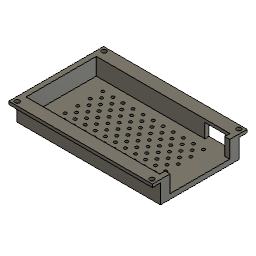
Portable+Battery+Case (Autodesk Fusion 360 design; units mm, degrees)
Autodesk Fusion 360 part; units mm, degrees
note: some values were not read from the file. Set by a fixed rule: which sketch regions a step uses.
sketch "Sketch1" plane through (0, 0, 0) normal (0, 1, 0) x (1, 0, 0)
  line L0 (-66.4, 34.9) -> (66.4, 34.9)
  line L1 (66.4, 34.9) -> (66.4, -34.9)
  line L2 (66.4, -34.9) -> (-66.4, -34.9)
  line L3 (-66.4, -34.9) -> (-66.4, 34.9)
  line L4 (-71.4, -39.15) -> (71.4, -39.15)
  line L5 (71.4, 39.15) -> (71.4, -39.15)
  line L6 (0, 0) -> (-71.6, 0) construction
  line L7 (-71.4, 39.15) -> (71.4, 39.15)
  line L8 (-71.4, 39.15) -> (-71.4, -39.15)
  dimension "d1" = 69.8
  dimension "d2" = 132.8
  dimension "d3" = 66.4
  dimension "d4" = 34.9
  dimension "d40" = 4.25
  dimension "d46" = 4.25
  dimension "d47" = 5
  dimension "d63" = 5
  constraint horizontal L0
  constraint vertical L1
  constraint horizontal L2
  constraint vertical L3
  constraint coincident L6.start origin
  constraint horizontal L6
  constraint perpendicular L5 L7
  constraint perpendicular L4 L5
  constraint perpendicular L7 L8
  measures "d1" distance of L0.start L2.end
  measures "d2" distance of L0.start L0.end
  measures "d3" distance of L6.start L3
  measures "d4" distance of L6.start L0
  measures "d40" distance of L2 L4
  measures "d46" distance of L0 L7
  measures "d47" distance of L1 L5
  measures "d63" distance of L3 L8
extrude "Extrude1" add sketch "Sketch1" along normal blind 5 contours L0 L1 L2 L3
extrude "Extrude2" add sketch "Sketch1" along normal blind 22.018
sketch "Sketch3" plane through (0, 22.018, 0) normal (0, 1, 0) x (-1, 0, 0)
  line L0 (-66.4, 34.9) -> (66.4, 34.9)
  line L1 (66.4, 34.9) -> (66.4, -34.9)
  line L2 (66.4, -34.9) -> (-66.4, -34.9)
  line L3 (-66.4, -34.9) -> (-66.4, 34.9)
  line L4 (62.4, -47.15) -> (-71.4, -47.15)
  line L5 (-71.4, -47.15) -> (-71.4, 47.15)
  line L6 (-71.4, 47.15) -> (71.4, 47.15)
  circle A0 centre (66.9, -43.15) radius 2.25
  circle A1 centre (-66.9, -43.15) radius 2.25
  circle A2 centre (-66.9, 43.15) radius 2.25
  circle A3 centre (66.9, 43.15) radius 2.25
  line L7 (71.4, 39.15) -> (-71.4, 39.15)
  line L8 (-71.4, 39.15) -> (-71.4, -39.15)
  line L9 (-71.4, -39.15) -> (71.4, -39.15)
  line L10 (62.4, -47.15) -> (71.4, -47.15)
  line L11 (71.4, 39.15) -> (71.4, 47.15)
  line L12 (71.4, -39.15) -> (71.4, 39.15)
  line L13 (71.4, -47.15) -> (71.4, -39.15)
  point P0 (-71.4, 0)
  point P1 (71.4, 39.15)
  dimension "d23" = 4.5
  dimension "d24" = 4
  dimension "d25" = 4.5
  dimension "d26" = 4.5
  dimension "d27" = 4
  dimension "d29" = 4.5
  dimension "d30" = 4.5
  dimension "d31" = 4
  dimension "d32" = 4.5
  dimension "d50" = 9
  dimension "d51" = 4.5
  dimension "d52" = 4
  dimension "d64" = 8
  dimension "d65" = 8
  dimension "d66" = 4.5
  constraint horizontal L4
  constraint vertical L5
  constraint horizontal L6
  constraint midpoint L5 P0
  constraint coincident L8.end L5
  constraint coincident P1 L7.start
  constraint perpendicular L6 L11
  constraint perpendicular L9 L13
  constraint coincident L9.end L12.start
  constraint perpendicular L10 L13
  measures "d23" diameter of A0
  measures "d24" distance of L4 A1.centre
  measures "d25" distance of L5 A1.centre
  measures "d26" diameter of A1
  measures "d27" distance of L6 A3.centre
  measures "d29" diameter of A3
  measures "d30" distance of L5 A2.centre
  measures "d31" distance of L6 A2.centre
  measures "d32" diameter of A2
  measures "d50" distance of L4.start L10.end
  measures "d51" distance of A3.centre L11
  measures "d52" distance of A0.centre L10
  measures "d64" distance of L6 L7
  measures "d65" distance of L10.end L9.end
  measures "d66" distance of A0.centre L13
extrude "Extrude4" add sketch "Sketch3" against normal blind 3 contours L4 L5 L9 L10 L13 | L5 L6 L7 L11
sketch "Sketch2" plane through (71.4, 0, 0) normal (1, 0, 0) x (0, 0, -1)
  line L0 (39.65, 0) -> (39.65, 18.75)
  line L1 (-34.65, 5) -> (34.65, 5)
  line L2 (34.65, 5) -> (-34.65, 5)
  line L3 (-29.65, 22.018) -> (29.65, 22.018)
  line L4 (29.65, 22.018) -> (29.65, 5)
  line L5 (29.65, 5) -> (-29.65, 5)
  line L6 (-29.65, 5) -> (-29.65, 22.018)
  line L7 (-39.15, 0) -> (39.15, 0)
  line L8 (39.15, 19.018) -> (47.15, 19.018)
  line L9 (47.15, 19.018) -> (47.15, 22.018)
  line L10 (47.15, 22.018) -> (-47.15, 22.018)
  line L11 (-47.15, 22.018) -> (-47.15, 19.018)
  line L12 (-47.15, 19.018) -> (-39.15, 19.018)
  line L13 (-39.15, 19.018) -> (-39.15, 0)
  line L14 (39.15, 0) -> (39.15, 19.018)
  point P0 (0, 22.018)
  dimension "d13" = 5
  dimension "d14" = 5
  constraint horizontal L3
  constraint vertical L4
  constraint horizontal L5
  constraint vertical L6
  constraint coincident L2 L4.end
  constraint midpoint L3 P0
  constraint coincident L10 P0
  measures "d13" distance of L1.start L6
  measures "d14" distance of L1.end L4
extrude "Extrude3" cut sketch "Sketch2" against normal up to surface (5 mm away) contours L1 L2 L3 L4 L5 L6 L10
sketch "Sketch6" plane through (0, 5, 0) normal (0, 1, 0) x (-1, 0, 0)
  line L0 (66.4, 34.9) -> (-66.4, 34.9)
  line L1 (-66.4, 34.9) -> (-66.4, 29.65)
  line L2 (-66.4, 29.65) -> (-71.4, 29.65)
  line L3 (-71.4, 29.65) -> (-71.4, -29.65)
  line L4 (-71.4, -29.65) -> (-66.4, -29.65)
  line L5 (-66.4, -29.65) -> (-66.4, -34.9)
  line L6 (-66.4, -34.9) -> (66.4, -34.9)
  line L7 (66.4, -34.9) -> (66.4, 34.9)
  circle A0 centre (0, 0) radius 1.5
  circle A1 centre (-50, -25) radius 1.5
  circle A2 centre (-40, -25) radius 1.5
  circle A3 centre (-30, -25) radius 1.5
  circle A4 centre (-20, -25) radius 1.5
  circle A5 centre (-10, -25) radius 1.5
  circle A6 centre (0, -25) radius 1.5
  circle A7 centre (10, -25) radius 1.5
  circle A8 centre (20, -25) radius 1.5
  circle A9 centre (30, -25) radius 1.5
  circle A10 centre (40, -25) radius 1.5
  circle A11 centre (50, -25) radius 1.5
  circle A12 centre (-50, -12.5) radius 1.5
  circle A13 centre (-40, -12.5) radius 1.5
  circle A14 centre (-30, -12.5) radius 1.5
  circle A15 centre (-20, -12.5) radius 1.5
  circle A16 centre (-10, -12.5) radius 1.5
  circle A17 centre (0, -12.5) radius 1.5
  circle A18 centre (10, -12.5) radius 1.5
  circle A19 centre (20, -12.5) radius 1.5
  circle A20 centre (30, -12.5) radius 1.5
  circle A21 centre (40, -12.5) radius 1.5
  circle A22 centre (50, -12.5) radius 1.5
  circle A23 centre (-50, 0) radius 1.5
  circle A24 centre (-40, 0) radius 1.5
  circle A25 centre (-30, 0) radius 1.5
  circle A26 centre (-20, 0) radius 1.5
  circle A27 centre (-10, 0) radius 1.5
  circle A28 centre (10, 0) radius 1.5
  circle A29 centre (20, 0) radius 1.5
  circle A30 centre (30, 0) radius 1.5
  circle A31 centre (40, 0) radius 1.5
  circle A32 centre (50, 0) radius 1.5
  circle A33 centre (-50, 12.5) radius 1.5
  circle A34 centre (-40, 12.5) radius 1.5
  circle A35 centre (-30, 12.5) radius 1.5
  circle A36 centre (-20, 12.5) radius 1.5
  circle A37 centre (-10, 12.5) radius 1.5
  circle A38 centre (0, 12.5) radius 1.5
  circle A39 centre (10, 12.5) radius 1.5
  circle A40 centre (20, 12.5) radius 1.5
  circle A41 centre (30, 12.5) radius 1.5
  circle A42 centre (40, 12.5) radius 1.5
  circle A43 centre (50, 12.5) radius 1.5
  circle A44 centre (-50, 25) radius 1.5
  circle A45 centre (-40, 25) radius 1.5
  circle A46 centre (-30, 25) radius 1.5
  circle A47 centre (-20, 25) radius 1.5
  circle A48 centre (-10, 25) radius 1.5
  circle A49 centre (0, 25) radius 1.5
  circle A50 centre (10, 25) radius 1.5
  circle A51 centre (20, 25) radius 1.5
  circle A52 centre (30, 25) radius 1.5
  circle A53 centre (40, 25) radius 1.5
  circle A54 centre (50, 25) radius 1.5
  line L8 (50, -25) -> (40, -25) construction
  line L9 (40, -25) -> (40, -12.5) construction
  line L10 (40, -12.5) -> (50, -12.5) construction
  line L11 (50, -12.5) -> (50, -25) construction
  line L12 (50, -18.75) -> (40, -18.75) construction
  line L13 (45, -25) -> (45, -12.5) construction
  circle A55 centre (45, -18.75) radius 1.5
  circle A56 centre (35, -18.75) radius 1.5
  circle A57 centre (25, -18.75) radius 1.5
  circle A58 centre (15, -18.75) radius 1.5
  circle A59 centre (5, -18.75) radius 1.5
  circle A60 centre (-5, -18.75) radius 1.5
  circle A61 centre (-15, -18.75) radius 1.5
  circle A62 centre (-25, -18.75) radius 1.5
  circle A63 centre (-35, -18.75) radius 1.5
  circle A64 centre (-45, -18.75) radius 1.5
  circle A65 centre (45, -6.25) radius 1.5
  circle A66 centre (35, -6.25) radius 1.5
  circle A67 centre (25, -6.25) radius 1.5
  circle A68 centre (15, -6.25) radius 1.5
  circle A69 centre (5, -6.25) radius 1.5
  circle A70 centre (-5, -6.25) radius 1.5
  circle A71 centre (-15, -6.25) radius 1.5
  circle A72 centre (-25, -6.25) radius 1.5
  circle A73 centre (-35, -6.25) radius 1.5
  circle A74 centre (-45, -6.25) radius 1.5
  circle A75 centre (45, 6.25) radius 1.5
  circle A76 centre (35, 6.25) radius 1.5
  circle A77 centre (25, 6.25) radius 1.5
  circle A78 centre (15, 6.25) radius 1.5
  circle A79 centre (5, 6.25) radius 1.5
  circle A80 centre (-5, 6.25) radius 1.5
  circle A81 centre (-15, 6.25) radius 1.5
  circle A82 centre (-25, 6.25) radius 1.5
  circle A83 centre (-35, 6.25) radius 1.5
  circle A84 centre (-45, 6.25) radius 1.5
  circle A85 centre (45, 18.75) radius 1.5
  circle A86 centre (35, 18.75) radius 1.5
  circle A87 centre (25, 18.75) radius 1.5
  circle A88 centre (15, 18.75) radius 1.5
  circle A89 centre (5, 18.75) radius 1.5
  circle A90 centre (-5, 18.75) radius 1.5
  circle A91 centre (-15, 18.75) radius 1.5
  circle A92 centre (-25, 18.75) radius 1.5
  circle A93 centre (-35, 18.75) radius 1.5
  circle A94 centre (-45, 18.75) radius 1.5
  dimension "d67" = 3
  dimension "d70" = 50
  dimension "d71" = 25
  dimension "d72" = 3
  dimension "d75" = -90
  dimension "d76" = 37.5
  constraint coincident A0.centre origin
  constraint horizontal L8
  constraint vertical L9
  constraint horizontal L10
  constraint vertical L11
  constraint coincident A21.centre L9.end
  constraint coincident A11.centre L8.start
  constraint midpoint L11 L12.start
  constraint midpoint L9 L12.end
  constraint midpoint L8 L13.start
  constraint midpoint L10 L13.end
  constraint midpoint L13 A55.centre
  measures "d67" diameter of A0
  measures "d72" diameter of A55
extrude "Extrude7" cut sketch "Sketch6" against normal up to surface (5 mm away) contours A0 | A1 | A2 | A3 | A4 | A5 | A6 | A7 | A8 | A9 | A10 | A11 | A12 | A13 | A14 | A15 | A16 | A17 | A18 | A19 | A20 | A21 | A22 | A23 | A24 | A25 | A26 | A27 | A28 | A29 | A30 | A31 | A32 | A33 | A34 | A35 | A36 | A37 | A38 | A39 | A40 | A41 | A42 | A43 | A44 | A45 | A46 | A47 | A48 | A49 | A50 | A51 | A52 | A53 | A54 | A55 | A56 | A57 | A58 | A59 | A60 | A61 | A62 | A63 | A64 | A65 | A66 | A67 | A68 | A69 | A70 | A71 | A72 | A73 | A74 | A75 | A76 | A77 | A78 | A79 | A80 | A81 | A82 | A83 | A84 | A85 | A86 | A87 | A88 | A89 | A90 | A91 | A92 | A93 | A94
sketch "Sketch7" plane through (0, 0, -39.15) normal (0, 0, -1) x (-1, 0, 0)
  line L0 (71.4, 19.018) -> (-71.4, 19.018)
  line L1 (-71.4, 19.018) -> (-71.4, 0)
  line L2 (-71.4, 0) -> (71.4, 0)
  line L3 (71.4, 0) -> (71.4, 19.018)
  line L4 (66.4, 5) -> (-66.4, 5)
  line L5 (-66.4, 5) -> (-66.4, 22.018)
  line L6 (-66.4, 22.018) -> (66.4, 22.018)
  line L7 (66.4, 22.018) -> (66.4, 5)
  line L8 (-61.4, 5) -> (-41.4, 5)
  line L9 (-41.4, 5) -> (-41.4, 19.018)
  line L10 (-41.4, 19.018) -> (-61.4, 19.018)
  line L11 (-61.4, 19.018) -> (-61.4, 5)
  dimension "d83" = 5
  dimension "d84" = 20
  constraint horizontal L8
  constraint vertical L9
  constraint horizontal L10
  constraint vertical L11
  constraint coincident L4 L8.start
  constraint coincident L0 L10.end
  measures "d83" distance of L5 L11
  measures "d84" distance of L8.start L8.end
extrude "Extrude8" cut sketch "Sketch7" against normal up to surface (4.25 mm away) contours L0 L4 L8 L9 L10 L11
fillet "Fillet1" [suppressed]
equation "d3 = d2 / 2"
equation "d4 = d1 / 2"
equation "d9 = 5 mm"
equation "d11 = d9 + 0.67 in"
equation "d14 = d13"
equation "d24 = d27"
equation "d25 = d30"
equation "d26 = d23"
equation "d27 = d64 / 2"
equation "d29 = d23"
equation "d31 = d27"
equation "d32 = d23"
equation "d46 = d40"
equation "d51 = d30"
equation "d52 = d27"
equation "d63 = d47"
equation "d65 = d64"
equation "d66 = d30"
equation "d72 = d67"
